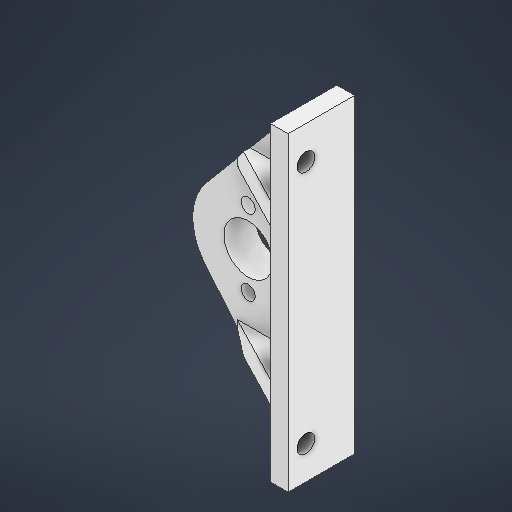
# Autodesk Inventor part: motor mount
Saved by Autodesk Inventor 2026.1 (Build 301233000, 233)
## iProperties
Created: 2024-09-27
Part Number: motor mount
Material: Generisch
Document SubType Name: Modeling
Designer: Familie Steib
Density: 1 g/cm^3
Appearance: Weiß
Author: Familie Steib
Autodesk Inventor part; units mm, degrees
sketch "Skizze1" plane through (0, 0, 0) normal (0, 0, 1) x (1, 0, 0)
  circle A0 centre (-17, 35) radius 12.5
  line L0 (0, 70) -> (0, 0)
  circle A1 centre (-17, 26.5) radius 1.6
  circle A2 centre (-17, 43.5) radius 1.6
  circle A3 centre (-17, 35) radius 5.5
  line L1 (3, 0) -> (0, 0)
  line L2 (0, 70) -> (-4, 70)
  line L3 (-4, 70) -> (-4, 0)
  line L4 (-4, 0) -> (0, 0)
  line L5 (0, 0) -> (0, 70)
  line L6 (-26.5845, 43.0242) -> (-4, 70)
  line L7 (-26.5845, 26.9758) -> (-4, 0)
  line L8 (0, 0) -> (-41.7952, 0)
  line L9 (-41.7952, 0) -> (-41.7952, 70)
  line L10 (-41.7952, 70) -> (0, 70)
  line L11 (0, 70) -> (0, 0)
  point P0 (0, 0)
  point P1 (0, 55)
  dimension "d0" = 25
  dimension "d2" = 8.5
  dimension "d3" = 17
  dimension "d6" = 3.2
  dimension "d7" = 3.2
  dimension "d8" = 11
  dimension "d10" = 70
  dimension "d11" = 17
  dimension "d23" = 4
  constraints: 24 end point, 4 centre point, 4 parallel, 2 horizontal, 2 perpendicular, 2 point on circle, 2 tangent, 1 coincident, 1 point on line
  measures "d0" diameter of A0
  measures "d2" distance of A0.centre A2.centre
  measures "d3" distance of A2.centre A1.centre
  measures "d6" diameter of A1
  measures "d7" diameter of A2
  measures "d8" diameter of A3
  measures "d10" distance of L0.start L0.end
  measures "d11" distance from line of L0 A0.centre
  measures "d23" distance of L4.end L3.end
extrude "Extrusion1" add sketch "Skizze1" along normal blind 7 contours A0 | A0 L6 L3 L7
ref_plane "Arbeitsebene1" through (0, 0, 39.5) normal (0, 0, 1) x (1, 0, 0)
extrude "Extrusion8" add sketch "Skizze1" along normal blind 15 contours L2 L0 L4 L3
ref_plane "Arbeitsebene2" through (-4, 50, 0) normal (0, 1, 0) x (1, 0, 0)
ref_plane "Arbeitsebene3" through (-4, 20, 0) normal (0, -1, 0) x (1, 0, 0)
sketch "Skizze8" plane through (-4, 50, 0) normal (0, 1, 0) x (1, 0, 0)
  line L0 (0, -15) -> (4, -15) projected
  line L1 (0, -15) -> (-15.5, -7)
  line L2 (-15.5, -7) -> (0, -7)
  line L3 (0, -7) -> (0, -15)
  line L4 (0, -7) -> (-22.5845, -7) projected
  point P0 (4, 0)
  dimension "d59" = 15.5
  constraints: 6 end point, 1 horizontal, 1 perpendicular, 1 point on line
  measures "d59" distance of L1.end L2.end
sketch "Skizze9" plane through (-4, 20, 0) normal (0, -1, 0) x (1, 0, 0)
  line L0 (0, 15) -> (-15.5, 7) projected
  line L1 (0, 7) -> (0, 15) projected
  line L2 (-15.5, 7) -> (0, 7) projected
  line L3 (-15.5, 7) -> (0, 15)
  line L4 (-22.5845, 7) -> (0, 7) projected
  line L5 (0, 7) -> (0, 15)
  line L6 (-15.5, 7) -> (0, 7)
  point P0 (4, 0)
  constraints: 6 end point, 2 perpendicular, 1 point on line
extrude "Extrusion9" add sketch "Skizze9" along normal blind 5
extrude "Extrusion10" add sketch "Skizze8" along normal blind 5
extrude "Extrusion11" cut sketch "Skizze1" along normal blind 20 contours A0 L7 L8 L9 L10 L6
sketch "Skizze10" plane through (-4, 0, 7) normal (-1, 0, 0) x (0, 0, 1)
  circle A0 centre (4, 7.5) radius 2
  circle A1 centre (4, 62.5) radius 2
  line L0 (0, 70) -> (8, 70) projected
  line L1 (1.5184, 55) -> (8, 55) projected
  line L2 (0, 0) -> (8, 0) projected
  line L3 (8, 15) -> (8, 0) projected
  line L4 (8, 70) -> (8, 55) projected
  line L5 (-7, 26.9758) -> (-7, 0) projected
  dimension "d67" = 4
  dimension "d68" = 4
  dimension "d69" = 7.5
  dimension "d71" = 7.5
  dimension "d72" = 4
  dimension "d73" = 4
  dimension "d76" = 11
  constraints: 2 centre point
  measures "d67" diameter of A1
  measures "d68" diameter of A0
  measures "d69" distance from line of L0 A1.centre
  measures "d71" distance from line of A0.centre L2
  measures "d72" distance from line of L3 A0.centre
  measures "d73" distance from line of L4 A1.centre
  measures "d76" distance from line of L5 A0.centre
extrude "Extrusion12" cut sketch "Skizze10" against normal blind 4
chamfer "Fase1" distance 2 angle 45 2 edges at (-18.6, 43.5, 0) (-18.6, 26.5, 0)
equation "\"d6\" = d7"
equation "\"d68\" = d67"
equation "\"d71\" = d69"
